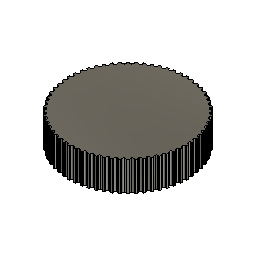
gear_64z (Autodesk Fusion 360 design; units mm, degrees)
Autodesk Fusion 360 part; units mm, degrees
sketch "Sketch1" plane through (0, 0, 0) normal (0, 0, 1) x (1, 0, 0) in component "gt2 pulley"
  circle A0 centre (0, 0) radius 20.3718 construction
  circle A1 centre (0, 0) radius 19.3678 construction
  line L0 (0, 0) -> (0, 20.3718) construction
  line L1 (0, 0) -> (0.9996, 20.3473) construction
  line L2 (0, 0) -> (1.4059, 20.3233) construction
  circle A2 centre (0, 0) radius 20.1178 construction
  arc A3 (0.3924, 19.9799) -> (0.4652, 19.6855) centre (1.3884, 20.0699) ccw
  circle A4 centre (0, 0) radius 19.9678 construction
  arc A5 (0.2448, 20.1163) -> (0, 20.1178) centre (0, 0) ccw
  arc A6 (0.3924, 19.9799) -> (0.2448, 20.1163) centre (0.2431, 19.9664) ccw
  arc A7 (0.4652, 19.6855) -> (0.9503, 19.3445) centre (0.9776, 19.8988) ccw
  arc A8 (0, 20.1178) -> (-0.2448, 20.1163) centre (0, 0) ccw
  arc A9 (-0.2448, 20.1163) -> (-0.3924, 19.9799) centre (-0.2431, 19.9664) ccw
  arc A10 (-0.4652, 19.6855) -> (-0.3924, 19.9799) centre (-1.3884, 20.0699) ccw
  arc A11 (-0.9504, 19.3445) -> (-0.4652, 19.6855) centre (-0.9776, 19.8988) ccw
  arc A12 (0.9503, 19.3445) -> (-0.9503, 19.3445) centre (0, 0) ccw
  point P0 (1.3884, 20.0699)
  point P1 (0, 20.1178)
  dimension "d18" = 40.7437
  dimension "d19" = 2.812
  dimension "d22" = 1.004
  dimension "d24" = 0.75
  dimension "d26" = 1
  dimension "d27" = 0.15
  dimension "d28" = 0.15
  dimension "d47" = 0.555
  dimension "d52" = 3.812
  constraint coincident A0.centre A1.centre
  constraint coincident A0 L0.end
  constraint vertical L0
  constraint coincident A0 L1.end
  constraint coincident A0 L2.end
  constraint concentric A1 A2
  constraint coincident A1 A7.end
  constraint coincident L1 A7.end
  constraint coincident A2 P0
  constraint coincident L2 P0
  constraint coincident P0 A3.centre
  constraint coincident A2 P1
  constraint coincident L0 P1
  constraint concentric A2 A4
  constraint coincident P1 A5.end
  constraint coincident A4 A6.centre
  constraint coincident A3.start A6.start
  constraint tangent A3 A6
  constraint tangent A3 A7
  constraint symmetric L0 A7.end A12.end
  constraint symmetric L0 A3.start A9.end
  constraint symmetric L0 A3.end A10.start
  constraint symmetric L0 A3 A10
  constraint symmetric L0 A5.start A8.end
  constraint symmetric L0 P1 A5.end
  constraint symmetric L0 A5 A8
  constraint symmetric L0 A6 A9
  constraint symmetric L0 A7 A11
  constraint coincident A1 A11.start
  constraint tangent A1 A7
  constraint coincident L1 A7.centre
  measures "d18" diameter of A0
  measures "d19" angle of L0 L1
  measures "d22" distance of A0 A1
  measures "d24" distance of A1 A2
  measures "d26" radius of A3
  measures "d27" distance of A2 A4
  measures "d28" radius of A6
  measures "d47" radius of A7
extrude "Extrude1" add sketch "Sketch1" along normal blind 10 makes body 1
pattern_circular "C-Pattern1" count 64 over 360 about axis through (0, 0, 1.75) along (0, 0, 1) of bodies 1 makes body 2 at (-1.1613, 19.333, 3.3333) makes body 3 at (-3.882, 18.9748, 6.6667) makes body 4 at (-6.3255, 18.3058, 6.6667) makes body 5 at (-6.7234, 18.1634, 3.3333) makes body 6 at (-8.4713, 17.4169, 3.3333) makes body 7 at (-10.1377, 16.5027, 3.3333) makes body 8 at (-11.7064, 15.4296, 3.3333) makes body 9 at (-13.1624, 14.2079, 3.3333) makes body 10 at (-14.4916, 12.8493, 3.3333) makes body 11 at (-16.1622, 10.6722, 6.6667) makes body 12 at (-16.72, 9.7753, 3.3333) makes body 13 at (-17.5976, 8.0893, 3.3333) makes body 14 at (-18.3058, 6.3255, 6.6667) makes body 15 at (-19.1261, 3.0506, 6.6667) makes body 16 at (-19.1881, 2.6327, 3.3333) makes body 17 at (-19.3537, 0.7393, 3.3333) makes body 18 at (-19.333, -1.1613, 3.3333) makes body 19 at (-18.9748, -3.882, 6.6667) makes body 20 at (-18.735, -4.9107, 3.3333) makes body 21 at (-17.8529, -7.5092, 6.6667) makes body 22 at (-16.72, -9.7753, 6.6667) makes body 23 at (-16.5027, -10.1377, 3.3333) makes body 24 at (-14.4916, -12.8493, 6.6667) makes body 25 at (-13.6202, -13.7696, 6.6667) makes body 26 at (-12.8493, -14.4916, 3.3333) makes body 27 at (-10.1377, -16.5028, 6.6667) makes body 28 at (-9.0366, -17.1304, 6.6667) makes body 29 at (-8.0893, -17.5976, 3.3333) makes body 30 at (-6.3255, -18.3058, 6.6667) makes body 31 at (-4.5008, -18.8376, 3.3333) makes body 32 at (-1.1613, -19.333, 6.6667) makes body 33 at (0.7393, -19.3537, 6.6667) makes body 34 at (1.1613, -19.333, 3.3333) makes body 35 at (4.5008, -18.8376, 6.6667) makes body 36 at (5.7232, -18.5029, 6.6667) makes body 37 at (7.5092, -17.8529, 6.6667) makes body 38 at (8.4713, -17.4169, 3.3333) makes body 39 at (10.8479, -16.0448, 6.6667) makes body 40 at (12.8493, -14.4916, 6.6667) makes body 41 at (13.7696, -13.6202, 6.6667) makes body 42 at (14.4916, -12.8493, 3.3333) makes body 43 at (16.1622, -10.6722, 6.6667) makes body 44 at (16.72, -9.7753, 3.3333) makes body 45 at (17.5976, -8.0893, 3.3333) makes body 46 at (18.3058, -6.3255, 3.3333) makes body 47 at (18.8376, -4.5008, 3.3333) makes body 48 at (19.1881, -2.6327, 3.3333) makes body 49 at (19.3537, -0.7393, 3.3333) makes body 50 at (19.333, 1.1613, 3.3333) makes body 51 at (19.1261, 3.0507, 3.3333) makes body 52 at (18.735, 4.9107, 3.3333) makes body 53 at (18.1634, 6.7234, 3.3333) makes body 54 at (17.4169, 8.4713, 3.3333) makes body 55 at (16.5027, 10.1377, 3.3333) makes body 56 at (14.4916, 12.8493, 6.6667) makes body 57 at (14.2079, 13.1624, 3.3333) makes body 58 at (12.8493, 14.4916, 3.3333) makes body 59 at (10.1377, 16.5028, 6.6667) makes body 60 at (9.0366, 17.1304, 6.6667) makes body 61 at (8.0893, 17.5976, 3.3333) makes body 62 at (6.3255, 18.3058, 3.3333) makes body 63 at (3.6748, 19.016, 6.6667) makes body 64 at (2.6327, 19.1881, 3.3333)
sketch "Sketch2" plane through (0, 0, 10) normal (0, 0, 1) x (-1, 0, 0)
  arc A0 (-8.0085, -18.3088) -> (-7.9244, -18.4914) centre (-7.8653, -18.3535) ccw
  arc A1 (-7.9244, -18.4914) -> (-7.472, -18.6788) centre (0, 0) ccw
  arc A2 (-7.472, -18.6788) -> (-7.2834, -18.6092) centre (-7.4162, -18.5395) ccw
  arc A3 (-7.1035, -18.3651) -> (-7.2834, -18.6092) centre (-6.3977, -19.0735) ccw
  arc A4 (-6.5248, -18.2357) -> (-7.1035, -18.3651) centre (-6.7118, -18.7582) ccw
  arc A5 (-8.2808, -17.5083) -> (-6.5248, -18.2357) centre (0, 0) ccw
  arc A6 (-7.9631, -18.009) -> (-8.2808, -17.5083) centre (-8.5181, -18.01) ccw
  arc A7 (-8.0085, -18.3088) -> (-7.9631, -18.009) centre (-8.9631, -18.0108) ccw
  circle A8 centre (0, 0) radius 19.3678
  constraint concentric A1 A8
extrude "Extrude2" add sketch "Sketch2" against normal blind 10 contours A5 A8 bodies 1 2 3 4 5 6 7 8 9 10 11 12 13 14 15 16 17 18 19 20 21 22 23 24 25 26 27 28 29 30 31 32 33 34 35 36 37 38 39 40 41 42 43 44 45 46 47 48 49 50 51 52 53 54 55 56 57 58 59 60 61 62 63 64
extrude "Extrude4" [suppressed] in component "gt2 pulley"
pattern_circular "C-Pattern7" [suppressed] in component "gt2 pulley"
extrude "Extrude3" [suppressed] in component "gt2 pulley"
pattern_circular "C-Pattern6" [suppressed] in component "gt2 pulley"
extrude "Extrude2'" [suppressed] in component "gt2 pulley"
pattern_circular "C-Pattern5" [suppressed] in component "gt2 pulley"
extrude "Extrude1'" [suppressed] in component "gt2 pulley"
pattern_circular "C-Pattern4" [suppressed] in component "gt2 pulley"
pattern_circular "C-Pattern3" [suppressed] in component "gt2 pulley"
pattern_circular "C-Pattern2" [suppressed] in component "gt2 pulley"
pattern_circular "C-Pattern1'" [suppressed] in component "gt2 pulley"
copy_body "Body->Comp1" [suppressed] in component "Component"
copy_body "Body->Comp2" [suppressed] in component "Component'"
copy_body "Body->Comp3" [suppressed] in component "Component''"
copy_body "Body->Comp4" [suppressed] in component "Component'''"
copy_body "Body->Comp5" [suppressed] in component "Component''''"
copy_body "Body->Comp6" [suppressed] in component "Component'''''"
copy_body "Body->Comp7" [suppressed] in component "Component''''''"
copy_body "Body->Comp8" [suppressed] in component "Component'''''''"
copy_body "Body->Comp9" [suppressed] in component "Component''''''''"
copy_body "Body->Comp10" [suppressed] in component "Component'''''''''"
copy_body "Body->Comp11" [suppressed] in component "Component''''''''''"
copy_body "Body->Comp12" [suppressed] in component "Component'''''''''''"
copy_body "Body->Comp13" [suppressed] in component "Component''''''''''''"
copy_body "Body->Comp14" [suppressed] in component "Component'''''''''''''"
copy_body "Body->Comp15" [suppressed] in component "Component''''''''''''''"
copy_body "Body->Comp16" [suppressed] in component "Component'''''''''''''''"
copy_body "Body->Comp17" [suppressed] in component "Component''''''''''''''''"
copy_body "Body->Comp18" [suppressed] in component "Component'''''''''''''''''"
copy_body "Body->Comp19" [suppressed] in component "Component''''''''''''''''''"
copy_body "Body->Comp20" [suppressed] in component "Component'''''''''''''''''''"
component "gt2 pulley" placed x (1, 0, 0) y (0, 1, 0) z (0, 0, 1) at (0, 0, 0)
equation "NumTeeth = 64" comment "min 20"
equation "ToothPitch = 2 mm"
equation "PullyDia = NumTeeth * ToothPitch / PI"
equation "ToothAng = ( ( 360 / NumTeeth ) * 1 deg )"
equation "TransOffsetAngle = ToothAng * 0.2"
equation "Sholulder_Radius = 0.15 mm"
equation "Root_Radius = 0.555 mm"
equation "TransRadius = 1 mm"
equation "ToolHeight = 0.75 mm"
equation "PLD = 0.254 mm"
equation "d18 = PullyDia"
equation "d19 = ToothAng / 2"
equation "d22 = PLD + ToolHeight"
equation "d24 = ToolHeight"
equation "d26 = TransRadius"
equation "d27 = Sholulder_Radius"
equation "d31 = NumTeeth"
equation "d33 = NumTeeth"
equation "d35 = NumTeeth"
equation "d37 = NumTeeth"
equation "d41 = NumTeeth"
equation "d45 = NumTeeth"
equation "d47 = Root_Radius"
equation "d50 = NumTeeth"
